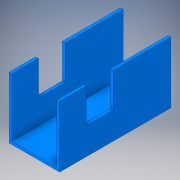
# Autodesk Inventor part: Hombro_base
Saved by Autodesk Inventor 2019 (Build 230136000, 136)
## iProperties
Created: 2020-02-08
Part Number: Hombro_base
Material: Generic
Document SubType Name: Modeling
Designer: Omar
Density: 1 g/cm^3
Appearance: Default
Author: Omar
Autodesk Inventor part; units mm, degrees
ref_plane "YZ Plane" through (0, 0, 0) normal (1, 0, 0) x (0, 1, 0)
ref_plane "XZ Plane" through (0, 0, 0) normal (0, 1, 0) x (-1, 0, 0)
ref_plane "XY Plane" through (0, 0, 0) normal (0, 0, 1) x (1, 0, 0)
sketch "Sketch1" plane through (0, 0, 0) normal (0, 1, 0) x (-1, 0, 0)
  line L0 (-25, 62.04) -> (25, 62.04)
  line L1 (25, 62.04) -> (25, -62.04)
  line L2 (25, -62.04) -> (-25, -62.04)
  line L3 (-25, -62.04) -> (-25, 62.04)
  line L4 (-25, 62.04) -> (25, -62.04) construction
  line L5 (25, 62.04) -> (-25, -62.04) construction
  circle A0 centre (0, 17.59) radius 5
  point P0 (0, 0)
  dimension "d0" = 50
  dimension "d1" = 124.08
  dimension "d2" = 10
  dimension "d3" = 44.45
  dimension "d4" = 25
  constraints: 12 end point, 2 midpoint, 2 parallel, 1 centre point, 1 horizontal, 1 perpendicular
  measures "d0" distance of L1.end L2.end
  measures "d1" distance of L0.end L1.end
  measures "d2" diameter of A0
  measures "d3" distance from line of L0 A0.centre
  measures "d4" distance from line of L1 A0.centre
extrude "Extrusion1" add sketch "Sketch1" along normal blind 3.18
sketch "Sketch4" plane through (0, 0, 0) normal (0, 1, 0) x (-1, 0, 0)
  circle A0 centre (0, 17.59) radius 5 projected
  line L0 (25, 62.04) -> (-25, 62.04) projected
  line L1 (-25, 62.04) -> (-25, -62.04) projected
  line L2 (-25, -62.04) -> (25, -62.04) projected
  line L3 (25, -62.04) -> (25, 62.04) projected
  line L4 (25, 62.04) -> (28.18, 62.04)
  line L5 (28.18, 62.04) -> (28.18, -62.04)
  line L6 (28.18, -62.04) -> (25, -62.04)
  line L7 (25, -62.04) -> (25, 62.04)
  line L8 (-25, 62.04) -> (-28.18, 62.04)
  line L9 (-28.18, 62.04) -> (-28.18, -62.04)
  line L10 (-28.18, -62.04) -> (-25, -62.04)
  line L11 (-25, -62.04) -> (-25, 62.04)
  point P0 (0, 0)
  dimension "d11" = 3.18
  dimension "d12" = 3.18
  constraints: 16 end point, 4 parallel, 2 horizontal, 2 perpendicular, 1 point on line
  measures "d11" distance of L5.end L6.end
  measures "d12" distance of L10.end L9.end
extrude "Extrusion3" add sketch "Sketch4" along normal blind 30 contours L4 L5 L6 L3 | L1 L10 L9 L8
sketch "Sketch5" plane through (0, 30, 0) normal (0, 1, 0) x (1, 0, 0)
  line L0 (-25, -62.04) -> (-25, 62.04) projected
  line L1 (-25, 62.04) -> (-28.18, 62.04) projected
  line L2 (-28.18, 62.04) -> (-28.18, -62.04) projected
  line L3 (-28.18, -62.04) -> (-25, -62.04) projected
  line L4 (25, -62.04) -> (28.18, -62.04) projected
  line L5 (28.18, -62.04) -> (28.18, 62.04) projected
  line L6 (28.18, 62.04) -> (25, 62.04) projected
  line L7 (25, 62.04) -> (25, -62.04) projected
  line L8 (-25, 62.04) -> (-25, -62.04) projected
  line L9 (-28.18, -62.04) -> (-25, -62.04)
  line L10 (-25, -62.04) -> (-25, -32.5)
  line L11 (-25, -32.5) -> (-28.18, -32.5)
  line L12 (-28.18, -32.5) -> (-28.18, -62.04)
  line L13 (-28.18, 62.04) -> (28.18, 62.04) projected
  line L14 (-28.18, 62.04) -> (-25, 62.04)
  line L15 (-25, 62.04) -> (-25, -2.5)
  line L16 (-25, -2.5) -> (-28.18, -2.5)
  line L17 (-28.18, -2.5) -> (-28.18, 62.04)
  line L18 (28.18, -62.04) -> (28.18, 62.04) projected
  line L19 (25, -62.04) -> (28.18, -62.04)
  line L20 (28.18, -62.04) -> (28.18, -32.5)
  line L21 (28.18, -32.5) -> (25, -32.5)
  line L22 (25, -32.5) -> (25, -62.04)
  line L23 (25, -62.04) -> (25, 62.04) projected
  line L24 (28.18, 62.04) -> (25, 62.04)
  line L25 (25, 62.04) -> (25, -2.5)
  line L26 (25, -2.5) -> (28.18, -2.5)
  line L27 (28.18, -2.5) -> (28.18, 62.04)
  point P0 (0, 0)
  dimension "d15" = 29.54
  dimension "d16" = 64.54
  dimension "d17" = 29.54
  dimension "d18" = 64.54
  constraints: 32 end point, 8 parallel, 4 horizontal, 4 perpendicular, 4 point on line
  measures "d15" distance of L10.end L9.end
  measures "d16" distance of L14.end L15.end
  measures "d17" distance of L20.end L19.end
  measures "d18" distance of L25.end L24.end
extrude "Extrusion4" add sketch "Sketch5" along normal blind 38.18 contours L3 L2 L11 L0 | L16 L2 L1 L0
sketch "Sketch6" plane through (0, 30, 0) normal (0, 1, 0) x (1, 0, 0)
  line L0 (25, -62.04) -> (28.18, -62.04) projected
  line L1 (28.18, -62.04) -> (28.18, 62.04) projected
  line L2 (28.18, 62.04) -> (25, 62.04) projected
  line L3 (25, 62.04) -> (25, -62.04) projected
  line L4 (28.18, -62.04) -> (28.18, 62.04) projected
  line L5 (25, -62.04) -> (25, 62.04) projected
  line L6 (28.18, -62.04) -> (25, -62.04)
  line L7 (25, -62.04) -> (25, -32.5)
  line L8 (25, -32.5) -> (28.18, -32.5)
  line L9 (28.18, -32.5) -> (28.18, -62.04)
  line L10 (28.18, 62.04) -> (25, 62.04)
  line L11 (25, 62.04) -> (25, -2.5)
  line L12 (25, -2.5) -> (28.18, -2.5)
  line L13 (28.18, -2.5) -> (28.18, 62.04)
  point P0 (0, 0)
  dimension "d21" = 29.54
  dimension "d22" = 64.54
  constraints: 16 end point, 4 parallel, 2 horizontal, 2 perpendicular, 2 point on line
  measures "d21" distance of L6.end L7.end
  measures "d22" distance of L11.end L10.end
extrude "Extrusion5" add sketch "Sketch6" along normal blind 38.18 contours L3 L8 L1 L0 | L3 L2 L1 L12
body "Solid1"
